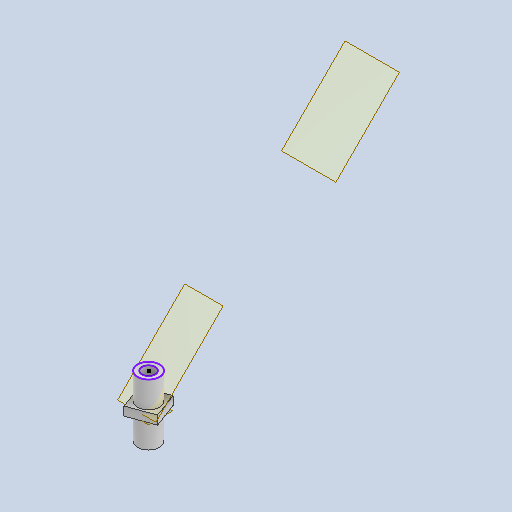
# Autodesk Inventor part: Part7
Saved by Autodesk Inventor 2025 (Build 290162000, 162)
## iProperties
Created: 2025-04-09
Part Number: Part7
Material: Generic
Document SubType Name: Modeling
Designer: Pravoslav
Density: 1 g/cm^3
Appearance: Default
Author: Pravoslav
Autodesk Inventor part; units mm, degrees
ref_plane "YZ Plane" through (0, 0, 0) normal (1, 0, 0) x (0, 1, 0)
ref_plane "XZ Plane" through (0, 0, 0) normal (0, 1, 0) x (-1, 0, 0)
ref_plane "XY Plane" through (0, 0, 0) normal (0, 0, 1) x (1, 0, 0)
sketch "Sketch1" plane through (0, 0, 0) normal (0, 1, 0) x (-1, 0, 0)
  circle A0 centre (0, 0) radius 0.75
  circle A1 centre (0, 0) radius 1.25
  dimension "d0" = 1.5
  dimension "d1" = 2.5
  constraints: 2 centre point, 2 coincident
  measures "d0" diameter of A0
  measures "d1" diameter of A1
extrude "Extrusion1" add sketch "Sketch1" along normal blind 2 and the other way blind 5
ref_plane "Work Plane1" through (0, -2, 0) normal (0, -1, 0) x (1, 0, 0)
sketch "Sketch2" plane through (0, -2, 0) normal (0, -1, 0) x (1, 0, 0)
  circle A0 centre (0, 0) radius 1.25
  circle A1 centre (0, 0) radius 0.75 projected
  line L0 (2.1326, -2.0398) -> (-2.1326, 2.0398) construction
  line L1 (-2.1326, -2.0398) -> (2.1326, 2.0398) construction
  line L2 (-1.9226, -0.8965) -> (0.8965, -1.9226)
  line L3 (0.8965, -1.9226) -> (1.9226, 0.8965)
  line L4 (1.9226, 0.8965) -> (-0.8965, 1.9226)
  line L5 (-0.8965, 1.9226) -> (-1.9226, -0.8965)
  line L6 (-1.9226, -0.8965) -> (1.9226, 0.8965) construction
  line L7 (0.8965, -1.9226) -> (-0.8965, 1.9226) construction
  line L8 (-1.9226, -0.8965) -> (1.0774, -0.8965) construction
  dimension "d18" = 3
  dimension "d19" = 20
  dimension "d20" = 3
  constraints: 18 end point, 4 midpoint, 2 parallel, 1 centre point, 1 coincident, 1 equal length, 1 horizontal, 1 perpendicular
  measures "d18" distance of L2.start L2.end
  measures "d19" angle of L2 L8
  measures "d20" distance of L3.end L2.end
extrude "Extrusion2" add sketch "Sketch2" against normal blind 1 contours A0 | A1 | L5 L4 L3 L2
ref_plane "Work Plane3" through (0, 2.4749, 2.4749) normal (0, 0.7071068, 0.7071068) x (1, 0, 0)
ref_plane "Work Plane2" through (0, 0, 0) normal (0, 0.7071068, 0.7071068) x (1, 0, 0)
sketch "Sketch6" plane through (0, 2, 0) normal (0, 1, 0) x (1, 0, 0)
  circle A0 centre (0, 0) radius 0.75
  circle A1 centre (0, 0) radius 1.25
  dimension "d10" = 1.5
  dimension "d11" = 2.5
  constraints: 2 centre point, 1 coincident
  measures "d10" diameter of A0
  measures "d11" diameter of A1
body "Solid1"
body "Solid2"
